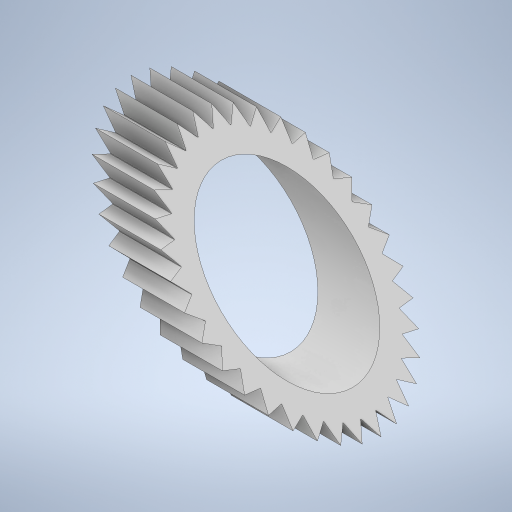
# Autodesk Inventor part: Test Gear
Saved by Autodesk Inventor 2023 (Build 270158030, 158C)
## iProperties
Created: 2022-09-20
Part Number: Test Gear
Material: Generic
Document SubType Name: Modeling
Designer: cjj5381
Density: 1 g/cm^3
Appearance: Default
Author: cjj5381
Autodesk Inventor part; units mm, degrees
ref_plane "YZ Plane" through (0, 0, 0) normal (1, 0, 0) x (0, 1, 0)
ref_plane "XZ Plane" through (0, 0, 0) normal (0, 1, 0) x (-1, 0, 0)
ref_plane "XY Plane" through (0, 0, 0) normal (0, 0, 1) x (1, 0, 0)
sketch "Sketch1" plane through (0, 0, 0) normal (1, 0, 0) x (0, 1, 0)
  circle A0 centre (0, 0) radius 11.8679
  line L0 (11.8205, 1.0604) -> (13.6572, 0)
  line L1 (13.6572, 0) -> (11.8205, -1.0604)
  line L2 (0, 0) -> (19.8155, 0) construction
  line L3 (11.4243, 3.2144) -> (13.4247, 2.5095)
  line L4 (13.4247, 2.5095) -> (11.8141, 1.1296)
  line L5 (10.6392, 5.2589) -> (12.735, 4.9336)
  line L6 (12.735, 4.9336) -> (11.4053, 3.2812)
  line L7 (9.4917, 7.1243) -> (11.6116, 7.1896)
  line L8 (11.6116, 7.1896) -> (10.6082, 5.3211)
  line L9 (8.021, 8.7471) -> (10.0928, 9.2008)
  line L10 (10.0928, 9.2008) -> (9.4498, 7.1797)
  line L11 (6.2772, 10.072) -> (8.2303, 10.8987)
  line L12 (8.2303, 10.8987) -> (7.9697, 8.7939)
  line L13 (4.3196, 11.0539) -> (6.0875, 12.2254)
  line L14 (6.0875, 12.2254) -> (6.2181, 10.1086)
  line L15 (2.2149, 11.6594) -> (3.7375, 13.1359)
  line L16 (3.7375, 13.1359) -> (4.2548, 11.079)
  line L17 (0.0347, 11.8679) -> (1.2601, 13.599)
  line L18 (1.2601, 13.599) -> (2.1466, 11.6722)
  line L19 (-2.1466, 11.6722) -> (-1.2601, 13.599)
  line L20 (-1.2601, 13.599) -> (-0.0347, 11.8679)
  line L21 (-4.2548, 11.079) -> (-3.7375, 13.1359)
  line L22 (-3.7375, 13.1359) -> (-2.2149, 11.6594)
  line L23 (-6.2181, 10.1086) -> (-6.0875, 12.2254)
  line L24 (-6.0875, 12.2254) -> (-4.3196, 11.0539)
  line L25 (-7.9697, 8.7939) -> (-8.2303, 10.8987)
  line L26 (-8.2303, 10.8987) -> (-6.2772, 10.072)
  line L27 (-9.4498, 7.1797) -> (-10.0928, 9.2008)
  line L28 (-10.0928, 9.2008) -> (-8.021, 8.7471)
  line L29 (-10.6082, 5.3211) -> (-11.6116, 7.1896)
  line L30 (-11.6116, 7.1896) -> (-9.4917, 7.1243)
  line L31 (-11.4053, 3.2812) -> (-12.735, 4.9336)
  line L32 (-12.735, 4.9336) -> (-10.6392, 5.2589)
  line L33 (-11.8141, 1.1296) -> (-13.4247, 2.5095)
  line L34 (-13.4247, 2.5095) -> (-11.4243, 3.2144)
  line L35 (-11.8205, -1.0604) -> (-13.6572, 0)
  line L36 (-13.6572, 0) -> (-11.8205, 1.0604)
  line L37 (-11.4243, -3.2144) -> (-13.4247, -2.5095)
  line L38 (-13.4247, -2.5095) -> (-11.8141, -1.1296)
  line L39 (-10.6392, -5.2589) -> (-12.735, -4.9336)
  line L40 (-12.735, -4.9336) -> (-11.4053, -3.2812)
  line L41 (-9.4917, -7.1243) -> (-11.6116, -7.1896)
  line L42 (-11.6116, -7.1896) -> (-10.6082, -5.3211)
  line L43 (-8.021, -8.7471) -> (-10.0928, -9.2008)
  line L44 (-10.0928, -9.2008) -> (-9.4498, -7.1797)
  line L45 (-6.2772, -10.072) -> (-8.2303, -10.8987)
  line L46 (-8.2303, -10.8987) -> (-7.9697, -8.7939)
  line L47 (-4.3196, -11.0539) -> (-6.0875, -12.2254)
  line L48 (-6.0875, -12.2254) -> (-6.2181, -10.1086)
  line L49 (-2.2149, -11.6594) -> (-3.7375, -13.1359)
  line L50 (-3.7375, -13.1359) -> (-4.2548, -11.079)
  line L51 (-0.0347, -11.8679) -> (-1.2601, -13.599)
  line L52 (-1.2601, -13.599) -> (-2.1466, -11.6722)
  line L53 (2.1466, -11.6722) -> (1.2601, -13.599)
  line L54 (1.2601, -13.599) -> (0.0347, -11.8679)
  line L55 (4.2548, -11.079) -> (3.7375, -13.1359)
  line L56 (3.7375, -13.1359) -> (2.2149, -11.6594)
  line L57 (6.2181, -10.1086) -> (6.0875, -12.2254)
  line L58 (6.0875, -12.2254) -> (4.3196, -11.0539)
  line L59 (7.9697, -8.7939) -> (8.2303, -10.8987)
  line L60 (8.2303, -10.8987) -> (6.2772, -10.072)
  line L61 (9.4498, -7.1797) -> (10.0928, -9.2008)
  line L62 (10.0928, -9.2008) -> (8.021, -8.7471)
  line L63 (10.6082, -5.3211) -> (11.6116, -7.1896)
  line L64 (11.6116, -7.1896) -> (9.4917, -7.1243)
  line L65 (11.4053, -3.2812) -> (12.735, -4.9336)
  line L66 (12.735, -4.9336) -> (10.6392, -5.2589)
  line L67 (11.8141, -1.1296) -> (13.4247, -2.5095)
  line L68 (13.4247, -2.5095) -> (11.4243, -3.2144)
  point P0 (11.8141, 1.1296)
  dimension "d0" = 60
  dimension "d3" = 360
  constraints: 138 end point, 1 coincident, 1 horizontal, 1 point on line, 1 symmetric about line, 175 other
  measures "d0" angle of L1 L0
extrude "Extrusion1" add sketch "Sketch1" along normal blind 50.8
sketch "Sketch2" plane through (0, 0, 0) normal (0, 0, 1) x (1, 0, 0)
  line L0 (-15.0129, 31.766) -> (41.9733, -25.2201)
  line L1 (-15.0129, 31.766) -> (65.5777, 31.766) construction
  line L2 (-6.0326, 31.766) -> (75.7664, -50.0331)
  line L3 (-15.0129, 31.766) -> (-15.0129, -18.6384)
  line L4 (-15.0129, -18.6384) -> (41.9733, -25.2201)
  line L5 (75.7664, -50.0331) -> (53.6248, 15.8173)
  line L6 (53.6248, 15.8173) -> (-6.0326, 31.766)
  point P0 (0, 0)
  dimension "d7" = 45
  dimension "d8" = 6.35
  constraints: 14 end point, 1 equal length, 1 horizontal, 1 parallel, 1 point on line, 1 vertical
  measures "d7" angle of L0 L1
  measures "d8" distance between parallel lines of L0 L2
extrude "Extrusion3" cut sketch "Sketch2" along normal mid plane 50.8
sketch "Sketch3" plane through (0, 0, 0) normal (1, 0, 0) x (0, 1, 0)
  circle A0 centre (0, 0) radius 9.525
  dimension "d15" = 19.05
  constraints: 1 centre point, 1 coincident
  measures "d15" diameter of A0
extrude "Extrusion4" cut sketch "Sketch3" along normal blind 50.8
body "Solid1"
